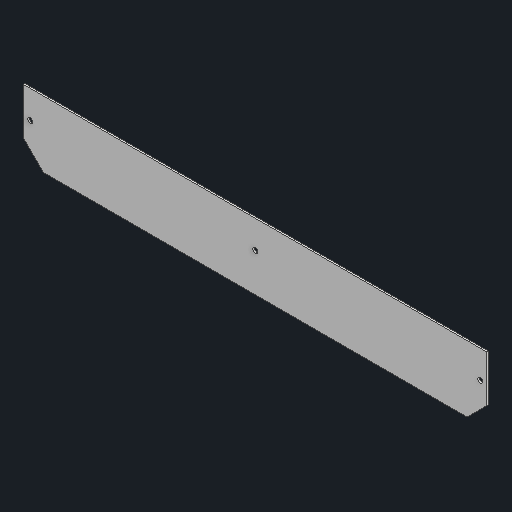
# Autodesk Inventor part: sideskirt
Saved by Autodesk Inventor 2023 (Build 270158000, 158)
## iProperties
Created: 2023-04-10
Part Number: sideskirt
Material: Generic
Document SubType Name: Modeling
Designer: Windows Macbook
Density: 1 g/cm^3
Appearance: Default
Author: Windows Macbook
Autodesk Inventor part; units mm, degrees
ref_plane "YZ Plane" through (0, 0, 0) normal (1, 0, 0) x (0, 1, 0)
ref_plane "XZ Plane" through (0, 0, 0) normal (0, 1, 0) x (-1, 0, 0)
ref_plane "XY Plane" through (0, 0, 0) normal (0, 0, 1) x (1, 0, 0)
sketch "Sketch1" plane through (0, 0, 0) normal (0, 0, 1) x (1, 0, 0)
  line L0 (444.5, 63.5) -> (0, 63.5)
  line L1 (444.5, 30.48) -> (487.6052, 30.48) construction
  line L2 (0, 63.5) -> (0, 19.05)
  line L3 (0, 19.05) -> (35.921, 19.05) construction
  line L4 (0, 19.05) -> (28.7368, 19.05) construction
  line L5 (444.5, 63.5) -> (444.5, 19.05)
  line L6 (444.5, 19.05) -> (425.45, 0)
  line L7 (0, 19.05) -> (19.05, 0)
  line L8 (0, 19.05) -> (26.9408, 19.05) construction
  line L9 (19.05, 0) -> (425.45, 0)
  point P0 (0, 0)
  dimension "d0" = 444.5
  dimension "d38" = 44.45
  dimension "d41" = 44.45
  dimension "d42" = 135
  dimension "d43" = 45
  constraints: 20 end point, 5 horizontal, 2 vertical, 1 equal length
  measures "d0" distance of L0.end L0.start
  measures "d38" distance of L0.end L2.end
  measures "d41" distance of L0.start L5.end
  measures "d42" angle of L5 L6
  measures "d43" angle of L7 L8
extrude "Extrusion1" add sketch "Sketch1" along normal blind 1.5875
sketch "Sketch2" plane through (0, 0, 1.5875) normal (0, 0, 1) x (1, 0, 0)
  line L0 (0.22, 63.5) -> (0.22, 50.8)
  line L1 (0.22, 50.8) -> (12.92, 63.5)
  line L2 (444.5, 63.5) -> (0, 63.5) projected
  line L3 (0, 63.5) -> (0, 30.48) projected
  line L4 (0, 63.5) -> (6.57, 57.15)
  line L5 (6.57, 57.15) -> (6.57, 49.53)
  line L6 (6.57, 57.15) -> (14.19, 57.15) construction
  line L7 (444.5, 30.48) -> (444.5, 63.5) projected
  line L8 (444.5, 63.5) -> (444.5, 50.8)
  line L9 (444.5, 50.8) -> (431.8, 63.5)
  line L10 (431.8, 63.5) -> (444.5, 63.5)
  line L11 (444.5, 63.5) -> (438.15, 57.15)
  line L12 (438.15, 57.15) -> (438.15, 49.53)
  line L13 (438.15, 49.53) -> (6.57, 49.53)
  line L14 (20.32, 0) -> (414.02, 0) projected
  line L15 (429.26, 15.24) -> (444.5, 0)
  line L16 (425.45, 0) -> (444.5, 19.05) projected
  line L17 (434.975, 9.525) -> (419.7086, -5.7414)
  line L18 (438.15, 49.53) -> (438.15, 24.13)
  line L19 (6.57, 49.53) -> (6.57, 24.13)
  line L20 (6.57, 49.53) -> (31.97, 49.53) construction
  line L21 (222.36, 49.53) -> (222.36, 36.83)
  point P0 (0, 0)
  point P1 (0, 30.48)
  point P2 (30.48, 0)
  point P3 (25.4, 0)
  point P4 (415.2184, 20.3013)
  point P5 (6.57, 36.83)
  point P6 (438.15, 36.83)
  dimension "d9" = 12.7
  dimension "d10" = 45
  dimension "d20" = 7.62
  dimension "d21" = 90
  dimension "d22" = 12.7
  dimension "d23" = 45
  dimension "d24" = 7.62
  dimension "d44" = 21.59
  dimension "d48" = 25.4
  dimension "d49" = 25.4
  dimension "d50" = 90
  constraints: 34 end point, 6 coincident, 5 midpoint, 5 vertical, 4 perpendicular, 3 point on line, 2 collinear, 2 horizontal, 1 other
  measures "d9" distance of L0.start L0.end
  measures "d10" angle of L1 L0
  measures "d20" distance of L4.end L5.end
  measures "d21" angle of L5 L6
  measures "d22" distance of L2.start L8.end
  measures "d23" angle of L8 L9
  measures "d24" distance of L11.end L12.end
  measures "d44" distance of L17.start L17.end
  measures "d48" distance of L18.start L18.end
  measures "d49" distance of L19.start L19.end
  measures "d50" angle of L19 L20
hole "Hole2" at (6.57, 36.83, 1.5875) at (222.36, 36.83, 1.5875) at (438.15, 36.83, 1.5875) direction (0, 0, -1) diameter 4.7625 end through all
body "Solid1"
